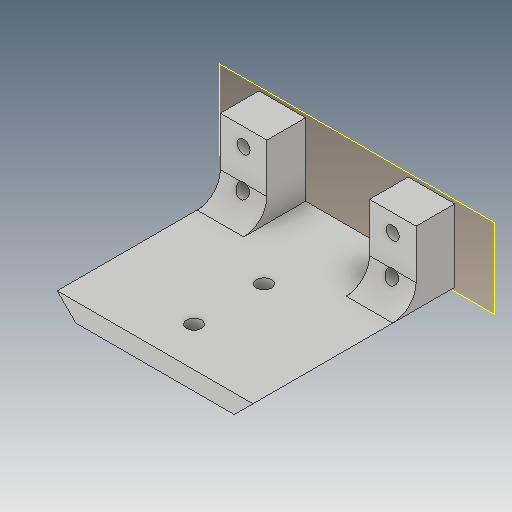
# Autodesk Inventor part: 31_MTP_wellplate_Solenoid_adapter
Saved by Autodesk Inventor 2019.4 (Build 234330000, 330)
## iProperties
Created: 2021-06-24
Part Number: 31_MTP_wellplate_Solenoid_adapter
Material: Generic
Document SubType Name: Modeling
Designer: diederichbenedict
Density: 1 g/cm^3
Appearance: Default
Author: diederichbenedict
Autodesk Inventor part; units mm, degrees
ref_plane "YZ Plane" through (0, 0, 0) normal (1, 0, 0) x (0, 1, 0)
ref_plane "XZ Plane" through (0, 0, 0) normal (0, 1, 0) x (-1, 0, 0)
ref_plane "Work Plane1" through (0, 0, 0) normal (0, 0, 1) x (1, 0, 0)
ref_plane "Work Plane2" through (40.2, -14.35, 43.3) normal (0, 0, 1) x (1, 0, 0)
sketch "Sketch1" plane through (0, 0, 0) normal (0, 0, 1) x (1, 0, 0)
  circle A0 centre (31.8, -10.75) radius 1.4 projected
  circle A1 centre (63.8, -10.75) radius 1.4 projected
  circle A2 centre (63.8, -2.75) radius 1.4 projected
  circle A3 centre (31.8, -2.75) radius 1.4 projected
  circle A4 centre (47.8, -6.75) radius 3.0846 projected
  line L0 (21, -14.5) -> (21, 1) projected
  line L1 (21, -14.5) -> (74.6, -14.5) projected
  line L2 (74.6, 1) -> (74.6, -14.5) projected
  line L3 (21, 1) -> (74.6, 1) projected
  circle A5 centre (47.8, -6.75) radius 2.196 construction
  line L4 (55.4, 0.85) -> (40.2, 0.85) construction
  line L5 (40.2, 0.85) -> (40.2, -14.35) construction
  line L6 (40.2, -14.35) -> (55.4, -14.35) construction
  line L7 (55.4, -14.35) -> (55.4, 0.85) construction
  line L8 (68.8, -14.5) -> (58.8, -14.5)
  line L9 (58.8, -14.5) -> (58.8, 1)
  line L10 (58.8, 1) -> (68.8, 1)
  line L11 (68.8, 1) -> (68.8, -14.5)
  line L12 (68.8, -14.5) -> (58.8, 1) construction
  line L13 (58.8, -14.5) -> (68.8, 1) construction
  line L14 (36.8, -14.5) -> (26.8, -14.5)
  line L15 (26.8, -14.5) -> (26.8, 1)
  line L16 (26.8, 1) -> (36.8, 1)
  line L17 (36.8, 1) -> (36.8, -14.5)
  line L18 (36.8, -14.5) -> (26.8, 1) construction
  line L19 (26.8, -14.5) -> (36.8, 1) construction
  line L20 (26.8, -14.5) -> (68.8, -14.5)
  line L21 (68.8, -14.5) -> (68.8, -18.5)
  line L22 (68.8, -18.5) -> (26.8, -18.5)
  line L23 (26.8, -18.5) -> (26.8, -14.5)
  point P0 (0, 0)
  point P1 (63.8, -6.75)
  point P2 (31.8, -6.75)
  dimension "d0" = 10
  dimension "d1" = 15.5
  dimension "d2" = 0
  dimension "d3" = 10
  dimension "d4" = 15.5
  dimension "d7" = 4
  constraints: 32 end point, 6 parallel, 4 midpoint, 3 horizontal, 3 perpendicular
  measures "d0" distance of L9.end L10.end
  measures "d1" distance of L8.end L9.end
  measures "d2" distance between parallel lines of L10 L3
  measures "d3" distance of L15.end L16.end
  measures "d4" distance of L14.end L15.end
  measures "d7" distance of L20.end L21.end
extrude "Extrusion1" add sketch "Sketch1" along normal up to surface (43.3 mm away) contours L15 L3 L17 L1 | L1 L21 L22 L23 | L9 L3 L11 L1
sketch "Sketch2" plane through (26.8, -18.5, 0) normal (0, -1, 0) x (1, 0, 0)
  circle A0 centre (20.9, 34.8462) radius 1 projected
  circle A1 centre (20.9, 19.8462) radius 1 projected
  line L0 (13.4, 13) -> (28.6, 13) projected
  line L1 (28.6, 13) -> (28.6, 43.3) projected
  line L2 (13.4, 43.3) -> (28.6, 43.3) projected
  line L3 (13.4, 13) -> (13.4, 43.3) projected
  point P0 (-26.8, 0)
hole "Hole1" at (47.7, -18.5, 19.8462) at (47.7, -18.5, 34.8462) direction (0, 1, 0) diameter 3.2 end through all
chamfer "Chamfer1" distance 4 angle 45 2 edges at (26.8, -18.5, 21.65) (68.8, -18.5, 21.65)
sketch "Sketch3" plane through (36.8, -14.5, 43.3) normal (0, 0, 1) x (1, 0, 0)
  line L0 (32, 0) -> (28, -4) projected
  line L1 (32, 15.5) -> (32, 0) projected
  line L2 (22, 15.5) -> (32, 15.5) projected
  line L3 (22, 0) -> (22, 15.5) projected
  line L4 (0, 0) -> (22, 0) projected
  line L5 (0, 15.5) -> (0, 0) projected
  line L6 (-10, 15.5) -> (0, 15.5) projected
  line L7 (-10, 0) -> (-10, 15.5) projected
  line L8 (-6, -4) -> (-10, 0) projected
  line L9 (28, -4) -> (-6, -4) projected
  circle A0 centre (27, 3.75) radius 1.4 projected
  circle A1 centre (27, 11.75) radius 1.4 projected
  circle A2 centre (-5, 3.75) radius 1.4 projected
  circle A3 centre (-5, 11.75) radius 1.4 projected
  line L10 (-10, 0) -> (32, 0)
  point P0 (-36.8, 14.5)
  constraints: 2 end point, 1 horizontal
extrude "Extrusion2" cut sketch "Sketch3" against normal blind 35 contours L10 L3 L2 L1 | L10 L7 L6 L5
fillet "Fillet1" radius 5 2 edges at (63.8, -14.5, 8.3) (31.8, -14.5, 8.3)
body "Solid1"
